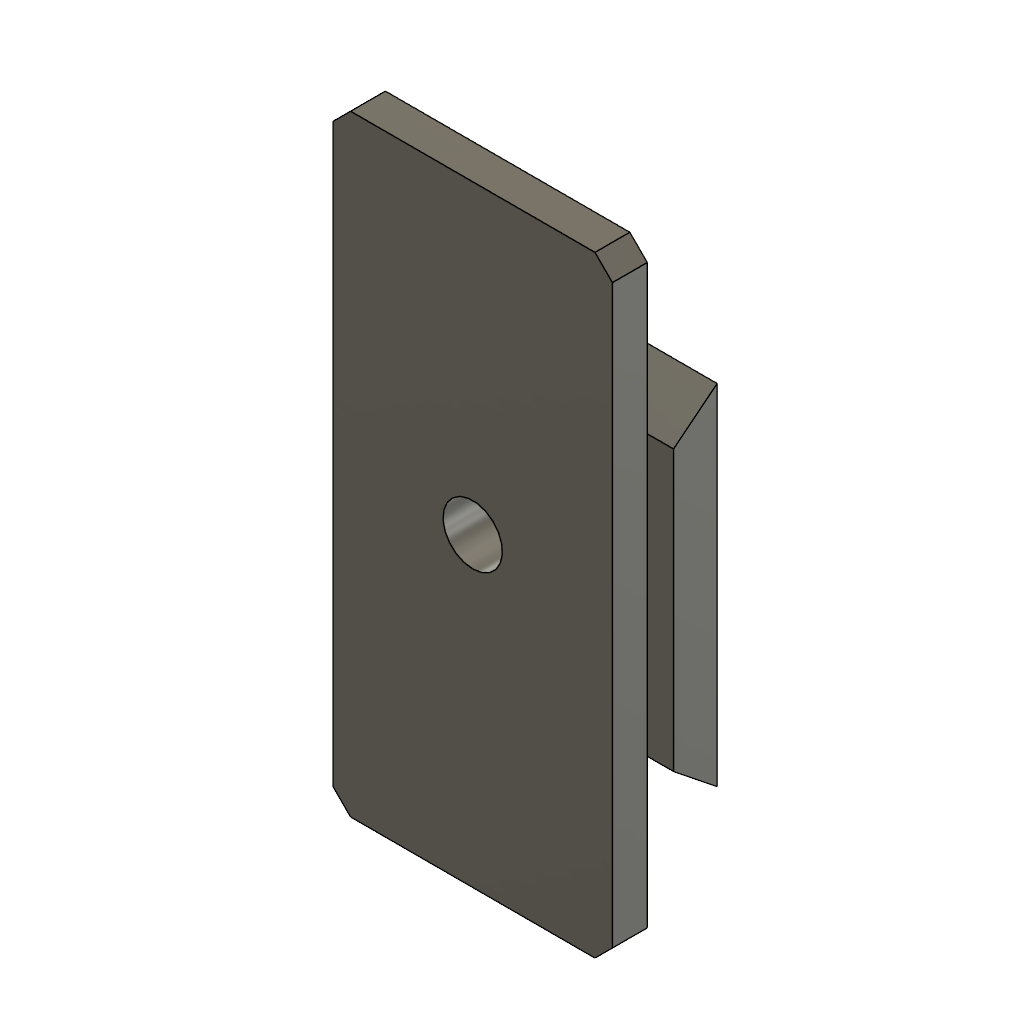
camera_plate (Autodesk Fusion 360 design; units mm, degrees)
part number: 2026-10-03-13-54-13-587
Autodesk Fusion 360 part; units mm, degrees
ref_plane "工作平面1" through (0, 0, 12.3) normal (0, 0, 1) x (1, 0, 0)
sketch "草图1" plane through (0, 0, 12.3) normal (0, 0, 1) x (1, 0, 0)
  line L0 (-33, -16) -> (33, -16)
  line L1 (33, -16) -> (35, -14)
  line L2 (35, -14) -> (35, 14)
  line L3 (35, 14) -> (33, 16)
  line L4 (33, 16) -> (-33, 16)
  line L5 (-33, 16) -> (-35, 14)
  line L6 (-35, 14) -> (-35, -14)
  line L7 (-35, -14) -> (-33, -16)
extrude "70 x 32 camera support plate" add sketch "草图1" along normal blind 4
ref_plane "工作平面2" through (0, 0, 7.3) normal (0, 0, 1) x (1, 0, 0)
sketch "草图2" plane through (0, 0, 7.3) normal (0, 0, 1) x (1, 0, 0)
  line L0 (-20, -19) -> (20, -19)
  line L1 (20, -19) -> (20, 19)
  line L2 (20, 19) -> (-20, 19)
  line L3 (-20, 19) -> (-20, -19)
ref_plane "工作平面3" through (0, 0, 12.3) normal (0, 0, 1) x (1, 0, 0)
sketch "草图3" plane through (0, 0, 12.3) normal (0, 0, 1) x (1, 0, 0)
  line L0 (-16, -19) -> (16, -19)
  line L1 (16, -19) -> (16, 19)
  line L2 (16, 19) -> (-16, 19)
  line L3 (-16, 19) -> (-16, -19)
loft "40 to 32 mm male dovetail" add profiles "草图2", "草图3" section 1 section 2
ref_plane "工作平面4" through (0, 0, 7.3) normal (0, 0, 1) x (1, 0, 0)
sketch "草图4" plane through (0, 0, 7.3) normal (0, 0, 1) x (1, 0, 0)
  circle A0 centre (0, 0) radius 3.4
extrude "1/4 inch metal screw clearance 6.8 mm" cut sketch "草图4" along normal blind 9
ref_plane "工作平面5" through (0, 0, 7.3) normal (0, 0, 1) x (1, 0, 0)
sketch "草图5" plane through (0, 0, 7.3) normal (0, 0, 1) x (1, 0, 0)
  circle A0 centre (0, 0) radius 7
extrude "14 x 3.5 mm screw head recess" cut sketch "草图5" along normal blind 3.5
move_body "Align camera long edge with gimbal arm - 90 degrees" bodies 1 to x (0, 1, 0) y (-1, 0, 0) z (0, 0, 1) at (0, 0, 0)
named bodies: "Camera_plate_1_4_optimized"
